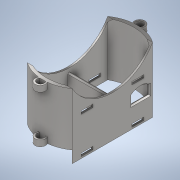
# Autodesk Inventor part: VR_Diş_Tasarım
Saved by Autodesk Inventor 2022 (Build 260153070, 153G)
## iProperties
Created: 2021-10-26
Part Number: VR_Diş_Tasarım
Material: Stainless Steel, Austenitic
Document SubType Name: Modeling
Designer: doguh
Density: 8 g/cm^3
Appearance: Semi-Polished
Author: doguh
## iProperties of the stored document VR_Diş_Tasarım_3DPrint.ipt
Created: 2021-10-26
Part Number: VR_Diş_Tasarım_3DPrint
Material: Generic
Document SubType Name: Modeling
Designer: doguh
Density: 1 g/cm^3
Appearance: Default
Author: doguh
Autodesk Inventor part; units mm, degrees
note: some values were not read from the file. Chosen so that the rebuilt part matches the saved one: second side of "ip_arka_dis".
ref_plane "YZ Plane" through (0, 0, 0) normal (1, 0, 0) x (0, 1, 0)
ref_plane "XZ Plane" through (0, 0, 0) normal (0, 1, 0) x (-1, 0, 0)
ref_plane "XY Plane" through (0, 0, 0) normal (0, 0, 1) x (1, 0, 0)
sketch "Sketch5" plane through (0, 0, 0) normal (0, 1, 0) x (-1, 0, 0)
  line L0 (38, 68) -> (38, -68)
  line L1 (-38, -68) -> (-38, 68)
  line L2 (-38, 68) -> (38, -68) construction
  line L3 (38, 68) -> (-38, -68) construction
  arc A0 (-38, -68) -> (38, -68) centre (0, -13.8333) ccw
  arc A1 (38, 68) -> (-38, 68) centre (0, 13.8333) ccw
  point P0 (0, 0)
  constraints: 8 end point, 4 point on circle, 2 centre point, 2 midpoint, 1 parallel
extrude "dis" add sketch "Sketch5" along normal blind 90
sketch "Sketch6" plane through (0, 90, 0) normal (0, 1, 0) x (1, 0, 0)
  line L0 (-35, -65) -> (-35, 65)
  line L1 (35, 65) -> (35, -65)
  line L2 (35, -65) -> (-35, 65) construction
  line L3 (-35, -65) -> (35, 65) construction
  arc A0 (-35, -65) -> (35, -65) centre (0, -1.4444) ccw
  arc A1 (35, 65) -> (-35, 65) centre (0, 1.4444) ccw
  point P0 (0, 0)
  dimension "d16" = 70
  dimension "d17" = 130
  constraints: 8 end point, 4 point on circle, 2 centre point, 2 midpoint, 1 parallel
  measures "d16" distance of L0.end L1.start
  measures "d17" distance of L0.start L0.end
extrude "ic" cut sketch "Sketch6" against normal blind 90
sketch "Sketch8" plane through (38, 0, 68) normal (1, 0, 0) x (0, 0, -1)
  line L0 (3, 90) -> (133, 90) projected
  line L1 (0, 0) -> (0, 90) projected
  line L2 (136, 0) -> (136, 90) projected
  arc A0 (0, 90) -> (136, 90) centre (68, 127.8) ccw
  line L3 (0, 90) -> (136, 90)
  line L4 (-6, 90) -> (3, 90) projected
  point P0 (68, 0)
  constraints: 2 end point, 2 point on circle, 1 centre point, 1 collinear
extrude "yarim_ay" cut sketch "Sketch8" against normal blind 90
sketch "Sketch10" plane through (38, 0, 68) normal (1, 0, 0) x (0, 0, -1)
  line L0 (136, 0) -> (151, 0) construction
  line L1 (131, 15) -> (101, 15)
  line L2 (101, 15) -> (101, 30)
  line L3 (131, 30) -> (131, 15)
  arc A0 (131, 30) -> (101, 30) centre (116, 10) ccw
  point P0 (68, 0)
  constraints: 8 end point, 2 horizontal, 2 point on circle, 1 centre point, 1 parallel, 1 perpendicular
extrude "parmak" cut sketch "Sketch10" against normal blind 3
chamfer "Chamfer1" distance 2 angle 45 4 edges at (38, 22.5, -33) (38, 22.5, -63) (38, 15, -48) (38, 35, -48)
sketch "Sketch11" plane through (38, 0, 68) normal (1, 0, 0) x (0, 0, -1)
  line L0 (0, 0) -> (-12, 0) projected
  line L1 (15, 45) -> (35, 45)
  line L2 (35, 45) -> (35, 50)
  line L3 (35, 50) -> (15, 50)
  line L4 (15, 50) -> (15, 45)
  line L5 (121, 45) -> (101, 45)
  line L6 (101, 45) -> (101, 50)
  line L7 (101, 50) -> (121, 50)
  line L8 (121, 50) -> (121, 45)
  point P0 (68, 0)
  point P1 (136, 0)
  constraints: 16 end point, 4 parallel, 2 horizontal, 2 perpendicular
extrude "sikigecme" cut sketch "Sketch11" against normal blind 3
sketch "Sketch12" plane through (0, 0, 0) normal (0, -1, 0) x (1, 0, 0)
  arc A0 (38, 68) -> (-38, 68) centre (0, 13.8333) ccw projected
  line L0 (35, 65) -> (35, -65)
  line L1 (38, -68) -> (38, 68)
  line L2 (38, 68) -> (35, 65)
  arc A1 (35, 65) -> (-35, 65) centre (0, 1.4444) ccw projected
  line L3 (38, -68) -> (35, -65)
  point P0 (0, 0)
  constraints: 8 end point, 2 point on circle, 2 point on line, 1 parallel, 1 perpendicular
extrude "telefon_tutucu" add sketch "Sketch12" along normal blind 20
sketch "Sketch13" plane through (38, 127.8, 0) normal (1, 0, 0) x (0, 0, -1)
  line L0 (-53, -144.8) -> (-33, -144.8)
  line L1 (-33, -144.8) -> (-33, -139.8)
  line L2 (-33, -139.8) -> (-53, -139.8)
  line L3 (-53, -139.8) -> (-53, -144.8)
  line L4 (53, -144.8) -> (33, -144.8)
  line L5 (33, -144.8) -> (33, -139.8)
  line L6 (33, -139.8) -> (53, -139.8)
  line L7 (53, -139.8) -> (53, -144.8)
  constraints: 16 end point, 4 parallel, 2 horizontal, 2 perpendicular
extrude "sikigecme2" cut sketch "Sketch13" against normal blind 3
sketch "Sketch15" plane through (-38, 0, -68) normal (-1, 0, 0) x (0, 0, 1)
  line L0 (121, -12) -> (121, -17) projected
  line L1 (121, 11) -> (101, 11)
  line L2 (101, 11) -> (101, 16)
  line L3 (101, 16) -> (121, 16)
  line L4 (121, 16) -> (121, 11)
  line L5 (15, -17) -> (15, -12) projected
  line L6 (15, 11) -> (35, 11)
  line L7 (35, 11) -> (35, 16)
  line L8 (35, 16) -> (15, 16)
  line L9 (15, 16) -> (15, 11)
  point P0 (68, 0)
  constraints: 16 end point, 4 parallel, 2 horizontal, 2 perpendicular
extrude "sikigecme3" cut sketch "Sketch15" against normal blind 3
sketch "Sketch16" plane through (35, 127.8, 0) normal (-1, 0, 0) x (0, 0, 1)
  line L0 (0, -127.8) -> (2.5, -127.8)
  line L1 (-65, -127.8) -> (65, -127.8) projected
  line L2 (0, -127.8) -> (0, -102.8)
  line L3 (2.5, -121.8) -> (-2.5, -121.8)
  line L4 (-2.5, -121.8) -> (-2.5, -83.8)
  line L5 (-2.5, -83.8) -> (2.5, -83.8)
  line L6 (2.5, -83.8) -> (2.5, -121.8)
  line L7 (2.5, -121.8) -> (-2.5, -83.8) construction
  line L8 (-2.5, -121.8) -> (2.5, -83.8) construction
  point P0 (-2.5, -127.8)
  dimension "d75" = 5
  dimension "d76" = 38
  constraints: 16 end point, 2 midpoint, 2 parallel, 1 horizontal, 1 perpendicular, 1 point on line, 1 vertical
  measures "d75" distance of L4.end L5.end
  measures "d76" distance of L3.end L4.end
extrude "orta_direk" add sketch "Sketch16" along normal blind 70
chamfer "Chamfer2" distance 2 angle 45 2 edges at (0, 44, -2.5) (0, 44, 2.5)
chamfer "Chamfer4" distance 2 angle 45 2 edges at (0, 6, -2.5) (0, 6, 2.5)
sketch "Sketch17" plane through (0, 0, 0) normal (0, -1, 0) x (1, 0, 0)
  arc A0 (-7.5, -79.5736) -> (7.5, -79.5736) centre (0, -84.192) ccw
  arc A1 (-7.5, -79.5736) -> (7.5, -79.5736) centre (0, -13.8333) ccw
  arc A2 (7.5, 79.5736) -> (-7.5, 79.5736) centre (0, 84.192) ccw
  arc A3 (7.5, 79.5736) -> (-7.5, 79.5736) centre (0, 13.8333) ccw
  point P0 (0, 0)
  point P1 (7.5, -79.5736)
  constraints: 8 point on circle, 4 centre point
extrude "ip_arka_dis" add sketch "Sketch17" against normal blind 10
sketch "Sketch19" plane through (0, 0, 0) normal (0, -1, 0) x (1, 0, 0)
  arc A0 (-5, -79.8108) -> (5, -79.8108) centre (0, -83.6786) ccw
  arc A1 (-7.5, -79.5736) -> (7.5, -79.5736) centre (0, -13.8333) ccw projected
  arc A2 (-5, -79.8108) -> (5, -79.8108) centre (0, -13.8333) ccw
  arc A3 (5, 79.8108) -> (-5, 79.8108) centre (0, 83.6786) ccw
  arc A4 (38, 68) -> (-38, 68) centre (0, 13.8333) ccw projected
  arc A5 (5, 79.8108) -> (-5, 79.8108) centre (0, 13.8333) ccw
  point P0 (0, 0)
  constraints: 12 point on circle, 4 centre point
extrude "ip_arka_ic" cut sketch "Sketch19" against normal blind 10
sketch "Sketch20" plane through (0, 90, 0) normal (0, 1, 0) x (1, 0, 0)
  arc A0 (7.5, 79.5736) -> (-7.5, 79.5736) centre (0, 84.192) ccw projected
  arc A1 (7.5, 79.5736) -> (-7.5, 79.5736) centre (0, 84.192) ccw
  arc A2 (38, 68) -> (7.5, 79.5736) centre (0, 13.8333) ccw projected
  arc A3 (7.5, 79.5736) -> (-7.5, 79.5736) centre (0, 13.8333) ccw
  arc A4 (-7.5, -79.5736) -> (7.5, -79.5736) centre (0, -84.192) ccw projected
  arc A5 (5, -79.8108) -> (7.5, -79.5736) centre (0, -13.8333) ccw projected
  arc A6 (-7.5, -79.5736) -> (7.5, -79.5736) centre (0, -84.192) ccw
  arc A7 (-38, -68) -> (-7.5, -79.5736) centre (0, -13.8333) ccw projected
  arc A8 (-7.5, -79.5736) -> (7.5, -79.5736) centre (0, -13.8333) ccw
  point P0 (0, 0)
  constraints: 8 point on circle, 4 centre point, 1 concentric
extrude "ip_on_dis" add sketch "Sketch20" against normal blind 10
sketch "Sketch21" plane through (0, 90, 0) normal (0, 1, 0) x (1, 0, 0)
  arc A0 (-5, -79.8108) -> (5, -79.8108) centre (0, -13.8333) ccw projected
  arc A1 (-5, -79.8108) -> (5, -79.8108) centre (0, -83.6786) ccw
  arc A2 (5, -79.8108) -> (7.5, -79.5736) centre (0, -13.8333) ccw projected
  arc A3 (-5, -79.8108) -> (5, -79.8108) centre (0, -13.8333) ccw
  arc A4 (7.5, 79.5736) -> (5, 79.8108) centre (0, 13.8333) ccw projected
  arc A5 (-5, 79.8108) -> (-7.5, 79.5736) centre (0, 13.8333) ccw projected
  arc A6 (5, 79.8108) -> (-5, 79.8108) centre (0, 83.6786) ccw
  arc A7 (5, 79.8108) -> (-5, 79.8108) centre (0, 13.8333) ccw
  point P0 (0, 0)
  constraints: 8 point on circle, 4 centre point
extrude "ip_on_ic" cut sketch "Sketch21" against normal blind 10
body "Solid2"
